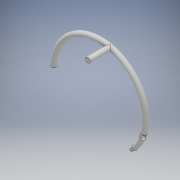
# Autodesk Inventor part: Ring
Saved by Autodesk Inventor 2018 (Build 220112000, 112)
## iProperties
Created: 2018-04-05
Part Number: Ring
Material: Generic
Document SubType Name: Modeling
Designer: anshs
Density: 1 g/cm^3
Appearance: Default
Mass: 9.95523 g
Surface Area: 60.5934 cm^2
Volume: 9.95523 cm^3
Author: anshs
Autodesk Inventor part; units mm, degrees
ref_plane "YZ Plane" through (0, 0, 0) normal (1, 0, 0) x (0, 1, 0)
ref_plane "XZ Plane" through (0, 0, 0) normal (0, 1, 0) x (-1, 0, 0)
sketch "Sketch1" plane through (0, 0, 0) normal (0, 0, 1) x (1, 0, 0)
  circle A0 centre (-61.5, 0) radius 3.35
  line L0 (0, -4.69) -> (0, 4.69) projected
  point P0 (0, 0)
  dimension "d0" = 6.7
  dimension "d2" = 61.5
  constraints: 1 centre point
  measures "d0" diameter of A0
  measures "d2" distance from line of L0 A0.centre
revolve "Revolution1" add sketch "Sketch1" angle 220 about axis through (0, -10, 0) along (0, 1, 0)
sketch "Sketch2" plane through (0, 0, 0) normal (0, 1, 0) x (-1, 0, 0)
  line L0 (-49.678, -41.6848) -> (-44.5455, -37.3781) projected
  line L1 (0, 0) -> (-76.6156, 91.3069) construction
  line L2 (-121.8781, 145.2487) -> (-43.4657, -70.1877) construction
  arc A0 (64.85, 0) -> (-49.678, -41.6848) centre (0, 0) ccw construction
  arc A1 (58.15, 0) -> (-44.5455, -37.3781) centre (0, 0) ccw construction
  line L3 (58.15, 0) -> (64.85, 0) projected
  circle A2 centre (-7.3644, 61.0575) radius 3.35
  line L4 (0, 0) -> (-12.8665, 72.9694) construction
  circle A3 centre (-13.9626, 59.894) radius 3.35
  point P0 (-60.9391, -22.18)
  dimension "d3" = 20
  dimension "d32" = 6.7
  dimension "d34" = 100
  dimension "d35" = 6.7
  constraints: 6 end point, 5 tangent, 2 centre point, 2 point on line, 1 perpendicular, 1 point on circle
  measures "d3" angle of L2 L1
  measures "d32" diameter of A2
  measures "d34" angle of L3 L4
  measures "d35" diameter of A3
ref_plane "Work Plane1" through (60.9391, 0, -22.18) normal (0.9397, 0, -0.342) x (0, 1, 0)
sketch "Sketch3" plane through (60.9391, 0, -22.18) normal (0.9397, 0, -0.342) x (0, 1, 0)
  line L0 (3, 5) -> (-3, 5)
  line L1 (-3, 5) -> (-3, -3)
  line L2 (-3, -3) -> (3, -3)
  line L3 (3, -3) -> (3, 5)
  point P0 (0, 0)
  dimension "d4" = 6
  dimension "d5" = 3
  dimension "d6" = 8
  dimension "d7" = 5
  constraints: 8 end point, 2 parallel, 1 horizontal, 1 perpendicular
  measures "d4" distance of L0.start L0.end
  measures "d5" distance from line of L1 point (0, 0)
  measures "d6" distance of L0.end L1.end
  measures "d7" distance from line of L0 point (0, 0)
extrude "Extrusion1" cut sketch "Sketch3" against normal blind 4.9
sketch "Sketch4" plane through (47.1117, 0, -39.5314) normal (-0.6428, 0, -0.766) x (-0.766, 0, 0.6428)
  line L0 (1.5, 2.5) -> (-1.5, 2.5)
  line L1 (-1.5, 2.5) -> (-1.5, -2.5)
  line L2 (-1.5, -2.5) -> (1.5, -2.5)
  line L3 (1.5, -2.5) -> (1.5, 2.5)
  circle A0 centre (0, 0) radius 3.35 projected
  point P0 (61.5, 0)
  dimension "d19" = 5
  dimension "d20" = 3
  dimension "d21" = 1.5
  dimension "d22" = 2.5
  constraints: 8 end point, 2 parallel, 1 horizontal, 1 perpendicular
  measures "d19" distance of L0.end L1.end
  measures "d20" distance of L1.end L2.end
  measures "d21" distance from line of L3 A0.centre
  measures "d22" distance from line of A0.centre L0
extrude "Extrusion2" add sketch "Sketch4" along normal blind 6 contours L3 L2 L1 L0
sketch "Sketch5" plane through (0, 0, 0) normal (0, 1, 0) x (-1, 0, 0)
  circle A0 centre (0, 0) radius 58 construction
  arc A1 (58.15, 0) -> (-44.5455, -37.3781) centre (0, 0) ccw construction
  circle A2 centre (0, 0) radius 65 construction
  dimension "d16" = 116
  dimension "d18" = 130
  constraints: 2 centre point, 1 coincident, 1 concentric
  measures "d16" diameter of A0
  measures "d18" diameter of A2
sketch "Sketch6" plane through (48.2608, -2.5, -40.4956) normal (0.766, 0, -0.6428) x (-0.6428, 0, -0.766)
  line L0 (0, 0) -> (0, 5) projected
  line L1 (0, 0) -> (6, 0) projected
  line L2 (6, 5) -> (6, 0) projected
  line L3 (0, 5) -> (6, 5) projected
  circle A0 centre (3, 2.5) radius 2
  point P0 (0, 2.5)
  dimension "d23" = 4
  dimension "d25" = 2.5
  dimension "d26" = 3
  constraints: 1 centre point
  measures "d23" diameter of A0
  measures "d25" distance from line of L1 A0.centre
  measures "d26" distance from line of L2 A0.centre
extrude "Extrusion3" cut sketch "Sketch6" against normal up to next contours A0
chamfer "Chamfer1" distance 1 angle 45 1 edges at (-64.85, 0, 0)
extrude "Extrusion4" add sketch "Sketch2" against normal blind 30 contours A3
body "Solid1"
